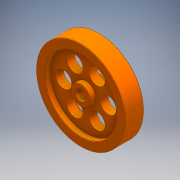
# Autodesk Inventor part: Volano
Saved by Autodesk Inventor 2016 (Build 200138000, 138)
## iProperties
Created: 2016-09-10
Part Number: Volano
Material: Generic
Document SubType Name: Modeling
Designer: Muhammad
Density: 1 g/cm^3
Appearance: Default
Author: Muhammad
Autodesk Inventor part; units mm, degrees
ref_plane "YZ Plane" through (0, 0, 0) normal (1, 0, 0) x (0, 1, 0)
ref_plane "XZ Plane" through (0, 0, 0) normal (0, 1, 0) x (-1, 0, 0)
ref_plane "XY Plane" through (0, 0, 0) normal (0, 0, 1) x (1, 0, 0)
sketch "Sketch1" plane through (0, 0, 0) normal (0, 1, 0) x (-1, 0, 0)
  circle A0 centre (0, 0) radius 40
  dimension "d0" = 80
  constraints: 1 centre point, 1 coincident
  measures "d0" diameter of A0
extrude "Extrusion1" add sketch "Sketch1" along normal mid plane 9
sketch "Sketch2" plane through (0, 4.5, 0) normal (0, 1, 0) x (1, 0, 0)
  line L0 (0, 0) -> (-25, 0) construction
  circle A0 centre (-25, 0) radius 9
  line L1 (0, -29.2747) -> (0, 26.9914) construction
  line L2 (0, 0) -> (29.6008, 0) construction
  circle A1 centre (25, 0) radius 9
  circle A2 centre (-12.5, -21.6506) radius 9
  circle A3 centre (12.5, -21.6506) radius 9
  circle A4 centre (25, 0) radius 9
  circle A5 centre (12.5, 21.6506) radius 9
  circle A6 centre (-12.5, 21.6506) radius 9
  dimension "d3" = 25
  dimension "d4" = 18
  dimension "d7" = 360
  constraints: 7 centre point, 6 end point, 2 horizontal, 1 coincident, 1 symmetric about line, 1 vertical, 14 other
  measures "d3" distance of L0.start L0.end
  measures "d4" diameter of A0
extrude "Extrusion2" cut sketch "Sketch2" against normal through all
sketch "Sketch3" plane through (0, 0, 0) normal (0, 1, 0) x (-1, 0, 0)
  circle A0 centre (0, 0) radius 11
  circle A1 centre (0, 0) radius 6
  constraints: 2 centre point, 2 coincident
extrude "Extrusion3" add sketch "Sketch3" along normal mid plane 21
sketch "Sketch4" plane through (0, 4.5, 0) normal (0, 1, 0) x (1, 0, 0)
  circle A0 centre (0, 0) radius 6
  constraints: 1 centre point, 1 coincident
extrude "Extrusion4" cut sketch "Sketch4" against normal through all
sketch "Sketch5" plane through (0, 4.5, 0) normal (0, 1, 0) x (1, 0, 0)
  point P0 (0, 0)
sketch "Sketch6" plane through (0, 0, 0) normal (0, 1, 0) x (-1, 0, 0)
  circle A0 centre (0, 0) radius 40
  circle A1 centre (0, 0) radius 50
  dimension "d17" = 100
  constraints: 2 centre point, 2 coincident
  measures "d17" diameter of A1
extrude "Extrusion5" add sketch "Sketch6" along normal mid plane 21
fillet "Fillet1" radius 0.5 6 edges at (40, 10.5, 0) (50, 10.5, 0) (40, -10.5, 0) (50, -10.5, 0) (11, 10.5, 0) (11, -10.5, 0)
body "Solid1"
